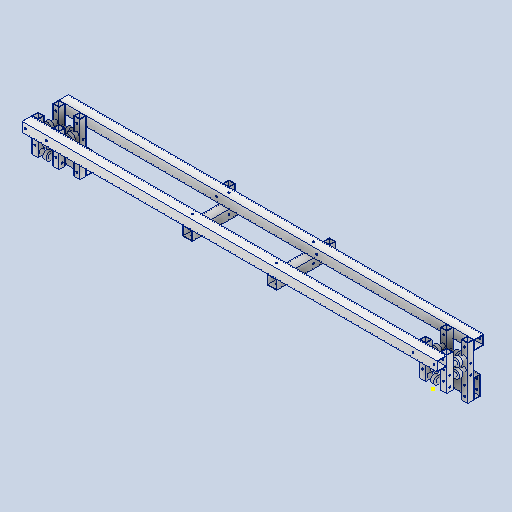
# Autodesk Inventor part: RZvector-Srunit-v3-ASP-Base
Saved by Autodesk Inventor 2025.2 (Build 292293000, 293)
## iProperties
Created: 2024-04-13
Part Number: RZvector-Srunit-v3-ASP-Base
Material: アルミニウム 6061
Document SubType Name: Modeling
Designer: haruy
Density: 2.7 g/cm^3
Appearance: アルミニウム - フラット
Author: haruy
Autodesk Inventor part; units mm, degrees
ref_plane "YZ Plane" through (0, 0, 0) normal (1, 0, 0) x (0, 1, 0)
ref_plane "XZ Plane" through (0, 0, 0) normal (0, 1, 0) x (-1, 0, 0)
ref_plane "XY Plane" through (0, 0, 0) normal (0, 0, 1) x (1, 0, 0)
derived "RZvector-Srunit-v2-Sketch-Base.ipt"
sketch "正面から" plane through (0, 0, 0) normal (0, 0, 1) x (1, 0, 0)
  line L0 (0, 0) -> (20, 0)
  line L1 (20, 0) -> (20, 80)
  line L2 (20, 80) -> (0, 80)
  line L3 (0, 80) -> (0, 0)
  line L4 (21.5, 92) -> (31.5, 92)
  line L5 (31.5, 92) -> (31.5, 0)
  line L6 (31.5, 0) -> (21.5, 0)
  line L7 (21.5, 0) -> (21.5, 92)
  line L8 (-11.5, 62) -> (-1.5, 62)
  line L9 (-1.5, 62) -> (-1.5, 0)
  line L10 (-1.5, 0) -> (-11.5, 0)
  line L11 (-11.5, 0) -> (-11.5, 62)
  line L12 (-1.5, 24.5) -> (21.5, 24.5)
  line L13 (21.5, 24.5) -> (21.5, 18.5)
  line L14 (21.5, 18.5) -> (-1.5, 18.5)
  line L15 (-1.5, 18.5) -> (-1.5, 24.5)
  line L16 (7.5, 28) -> (12.5, 28)
  line L17 (12.5, 28) -> (12.5, 15)
  line L18 (12.5, 15) -> (7.5, 15)
  line L19 (7.5, 15) -> (7.5, 28)
  circle A0 centre (26.5, 29.5) radius 3
  line L20 (31.5, 15) -> (-189.7387, 15)
  line L21 (-189.7387, 15) -> (-189.7387, 0)
  line L22 (-189.7387, 0) -> (31.5, 0)
  line L23 (31.5, 0) -> (31.5, 15)
  line L24 (31.5, 92) -> (41.5, 92)
  line L25 (41.5, 92) -> (41.5, 62)
  line L26 (41.5, 62) -> (31.5, 62)
  line L27 (31.5, 62) -> (31.5, 92)
  circle A1 centre (26.5, 29.5) radius 6.5
  circle A2 centre (-6.5, 29.5) radius 6.5
  line L28 (21.5, 23) -> (31.5, 23)
  line L29 (21.5, 20) -> (31.5, 20)
  circle A3 centre (26.5, 29.5) radius 1.5
  circle A4 centre (-6.5, 29.5) radius 3
  circle A5 centre (-6.5, 29.5) radius 1.5
  line L30 (-1.5, 40.5) -> (21.5, 40.5)
  line L31 (21.5, 40.5) -> (21.5, 34.5)
  line L32 (21.5, 34.5) -> (-1.5, 34.5)
  line L33 (-1.5, 34.5) -> (-1.5, 40.5)
  line L34 (7.5, 44) -> (12.5, 44)
  line L35 (12.5, 44) -> (12.5, 31)
  line L36 (12.5, 31) -> (7.5, 31)
  line L37 (7.5, 31) -> (7.5, 44)
  circle A6 centre (-6.5, 45.5) radius 6.5
  circle A7 centre (-6.5, 45.5) radius 3
  circle A8 centre (-6.5, 45.5) radius 1.5
  line L38 (-11.5, 62) -> (31.5, 62)
  line L39 (31.5, 62) -> (31.5, 52)
  line L40 (31.5, 52) -> (-11.5, 52)
  line L41 (-11.5, 52) -> (-11.5, 62)
  circle A9 centre (26.5, 45.5) radius 6.5
  circle A10 centre (26.5, 45.5) radius 3
  circle A11 centre (26.5, 45.5) radius 1.5
  line L42 (31.5, 47) -> (31.5, 62)
  line L43 (-145, 64.5) -> (31.5, 64.5)
  line L44 (31.5, 64.5) -> (31.5, 49.5)
  line L45 (31.5, 49.5) -> (-145, 49.5)
  line L46 (-145, 49.5) -> (-145, 64.5)
  line L47 (31.5, 52) -> (-295, 52)
  line L48 (-295, 52) -> (-295, 67)
  line L49 (-295, 67) -> (31.5, 67)
  line L50 (31.5, 67) -> (31.5, 52)
  line L51 (-11.5, 15) -> (31.5, 15)
  line L52 (31.5, 15) -> (31.5, -15)
  line L53 (31.5, -15) -> (-11.5, -15)
  line L54 (-11.5, -15) -> (-11.5, 15)
  line L55 (21.5, 0) -> (21.5, -15)
  line L56 (-1.5, 0) -> (-1.5, -15)
  line L57 (-1.5, 62) -> (-1.5, 67)
  line L58 (-11.5, 62) -> (-11.5, 67)
  point P0 (-6.5, 7.5)
  point P1 (26.5, 7.5)
  point P2 (-6.5, 59.5)
  point P3 (10, 57)
  point P4 (26.5, 59.5)
  point P5 (-1.5, 52)
  point P6 (-1.5, 62)
  point P7 (-135, 56.75)
  point P8 (-1.5, 49.5)
  point P9 (-1.5, 49.6533)
  point P10 (-1.3765, 49.5)
  point P11 (-6.5, -7.5)
  point P12 (26.5, -7.5)
  point P13 (31.5, 0)
  point P14 (21.5, 67)
  point P15 (31.5, 67)
  point P16 (21.5, 15)
  point P17 (31.5, 0)
  point P18 (-1.5, 15)
  dimension "d1" = 7.5
  dimension "d2" = 7.5
  dimension "d3" = 5
  dimension "d4" = 5
  dimension "d6" = 5
  dimension "d7" = 10
  dimension "d8" = 5
  dimension "d10" = 5
  dimension "d90" = 176.5
  dimension "d91" = 15
  dimension "d92" = 2.5
  dimension "d93" = 0
  dimension "d94" = 7.25
  dimension "d95" = 10
  dimension "d179" = 15
  dimension "d180" = 326.5
  dimension "d181" = 7.5
  dimension "d182" = 7.5
  dimension "d183" = 43
  dimension "d184" = 30
  measures "d1" distance from line of point (-6.5, 7.5) L10
  measures "d2" distance from line of point (26.5, 7.5) L6
  measures "d3" distance from line of point (-6.5, 7.5) L9
  measures "d4" distance from line of point (26.5, 7.5) L7
  measures "d6" distance from line of point (-6.5, 59.5) L9
  measures "d7" distance from line of point (10, 57) L3
  measures "d8" distance from line of point (10, 57) L40
  measures "d10" distance from line of point (26.5, 59.5) L5
  measures "d90" distance of L44.end L45.end
  measures "d91" distance of L43.end L44.end
  measures "d92" distance between parallel lines of L8 L43
  measures "d93" distance between parallel lines of L5 L44
  measures "d94" distance from line of point (-135, 56.75) L45
  measures "d95" distance from line of L46 point (-135, 56.75)
  measures "d179" distance of L47.end L48.end
  measures "d180" distance between parallel lines of L27 L48
  measures "d181" distance from line of point (-6.5, 59.5) L47
  measures "d182" distance from line of point (26.5, 59.5) L40
  measures "d183" distance of L52.end L53.end
  measures "d184" distance of L51.end L52.end
sketch "横から" plane through (0, 0, 0) normal (1, 0, 0) x (0, 1, 0)
  line L0 (0, 0) -> (200, 0)
  line L1 (200, 0) -> (200, -20)
  line L2 (200, -20) -> (0, -20)
  line L3 (0, -20) -> (0, 0)
  circle A0 centre (21.5, 6.5) radius 6.5
  circle A1 centre (21.5, -26.5) radius 6.5
  line L4 (15, 26.5) -> (0, 26.5)
  line L5 (0, 26.5) -> (0, 11.5)
  line L6 (0, 11.5) -> (15, 11.5)
  line L7 (15, 11.5) -> (15, 26.5)
  line L8 (15, -31.5) -> (0, -31.5)
  line L9 (0, -31.5) -> (0, -46.5)
  line L10 (0, -46.5) -> (15, -46.5)
  line L11 (15, -46.5) -> (15, -31.5)
  line L12 (62, 11.5) -> (0, 11.5)
  line L13 (0, 11.5) -> (0, 1.5)
  line L14 (0, 1.5) -> (62, 1.5)
  line L15 (62, 1.5) -> (62, 11.5)
  line L16 (62, -21.5) -> (0, -21.5)
  line L17 (0, -21.5) -> (0, -31.5)
  line L18 (0, -31.5) -> (62, -31.5)
  line L19 (62, -31.5) -> (62, -21.5)
  line L20 (36, -7.5) -> (23, -7.5)
  line L21 (23, -7.5) -> (23, -12.5)
  line L22 (23, -12.5) -> (36, -12.5)
  line L23 (36, -12.5) -> (36, -7.5)
  line L24 (92, 11.5) -> (62, 11.5)
  line L25 (62, 11.5) -> (62, -31.5)
  line L26 (62, -31.5) -> (92, -31.5)
  line L27 (92, -31.5) -> (92, 11.5)
  circle A2 centre (37.5, 6.5) radius 6.5
  circle A3 centre (37.5, -26.5) radius 6.5
  line L28 (52, -7.5) -> (39, -7.5)
  line L29 (39, -7.5) -> (39, -12.5)
  line L30 (39, -12.5) -> (52, -12.5)
  line L31 (52, -12.5) -> (52, -7.5)
  line L32 (52, 11.5) -> (52, -31.5)
  point P0 (62, -26.5)
extrude "押し出し1" add sketch "正面から" along normal blind 10 contours L10 L11 L20 L9 | L20 L11 A2 L9 | L11 A2 L9 | A2 L11 A6 L9 | L11 L45 L9 A6 | L11 A6 L9 L45 | L11 L40 A6 | A6 L40 L9 | L11 L8 L9 L40 | A4 | A5 | A7 | A8
extrude "押し出し2" add sketch "正面から" along normal blind 10 separate body contours L7 L20 L5 L6 | L7 L29 L5 L20 | L7 A1 L28 | L7 L28 L5 L29 | A1 L5 L7 | L7 A9 L5 A1 | L28 A1 L5 | A9 L7 L45 L5 | A9 L5 L45 L7 | L7 L40 A9 | A9 L40 L5 | L7 L38 L5 L40 | L7 L43 L5 L38 | L7 L49 L5 L43 | L7 L4 L5 L49 | A0 | A3 | A10 | A11
ref_plane "作業平面1" through (-1.5, 0, -23) normal (0, 0, -1) x (-1, 0, 0)
extrude "押し出し3" add sketch "正面から" against normal blind 10 from surface at -23 separate body contours L10 L11 L20 L9 | L20 L11 A2 L9 | L11 A2 L9 | A2 L11 A6 L9 | L11 L45 L9 A6 | L11 A6 L9 L45 | L11 L40 A6 | A6 L40 L9 | A4 | A5 | A7 | A8
extrude "押し出し4" add sketch "正面から" against normal blind 10 from surface at -23 separate body contours L7 L20 L5 L6 | L7 L29 L5 L20 | L7 A1 L28 | L7 L28 L5 L29 | A1 L5 L7 | L7 A9 L5 A1 | L28 A1 L5 | A9 L7 L45 L5 | A9 L5 L45 L7 | L7 L40 A9 | A9 L40 L5 | L7 L38 L5 L40 | L7 L43 L5 L38 | L7 L49 L5 L43 | L7 L4 L5 L49 | A0 | A3 | A10 | A11
ref_plane "作業平面2" through (-11.5, 0, 10) normal (0, 0, 1) x (1, 0, 0)
extrude "押し出し5" add sketch "正面から" along normal blind 15 from surface at 10 separate body contours L45 A6 L11 | L11 A6 L9 L45 | L45 L46 L47 L11 A6 | L45 A6 L9 L40 L3 | L3 L40 L1 L45 | L45 L9 A6 | L11 L40 A6 | L1 L40 L7 A9 L45 | A9 L7 L45 | L40 L9 L38 L3 | L3 L38 L1 L40 | A6 L40 L9 | L47 L46 L43 L58 L11 | L11 L8 L9 L40 | L1 L38 L7 L40 | A9 L5 L45 L7 | L7 L40 A9 | A9 L40 L5 | L38 L57 L43 L3 | L3 L43 L1 L38 | L58 L43 L57 L8 | L1 L43 L7 L38 | L7 L38 L5 L40 | L7 L43 L5 L38 picked at (-11.5139, 49.5853) picked at (-6.5, 50.3333) picked at (-1.4861, 49.5853) picked at (21.4861, 49.5853) picked at (26.5, 50.3333)
sketch "スケッチ3" plane through (31.5, 0, 0) normal (1, 0, 0) x (0, 0, -1)
  line L0 (-10, 92) -> (-10, 0) projected
  line L1 (-10, 92) -> (33, 92)
  line L2 (33, 92) -> (33, 62)
  line L3 (33, 62) -> (-10, 62)
  line L4 (-10, 62) -> (-10, 92)
  point P0 (0, 0)
  dimension "d23" = 43
  dimension "d24" = 30
  constraints: 8 end point, 2 parallel, 1 horizontal, 1 perpendicular
  measures "d23" distance of L2.end L3.end
  measures "d24" distance of L1.end L2.end
extrude "押し出し6" add sketch "スケッチ3" along normal blind 10 separate body
shell "シェル1" thickness 1 removed faces 11 at (-4.8333, 52, -26.3333) at (-8.1667, 0, -26.3333) at (24.8333, 0, -26.3333) at (-8.1667, 0, 3.3333) at (24.8333, 0, 3.3333) at (31.5, 54.5, 20) at (28.1667, 92, 6.6667) at (28.1667, 92, -26.3333) at (38.1667, 72, 10) at (34.8333, 72, -33) at (-4.8333, 62, 3.3333) bodies 3 4 1 2 5 6
hole "穴1" at (-6.5, 7.5, 0) at (26.5, 7.5, 0) at (-6.5, 59.5, 0) at (10, 57, 0) at (26.5, 59.5, 0) at (26.5, 29.5, 0) at (-6.5, 29.5, 0) at (-6.5, 45.5, 0) at (26.5, 45.5, 0) at (-135, 56.75, 0) direction (0, 0, 1) diameter 3 end through all both bodies 2 1 5 3
hole "穴2" at (26.5, 45.5, 0) at (26.5, 29.5, 0) at (26.5, 7.5, 0) direction (0, 0, -1) diameter 3 end through all bodies 4
sketch "スケッチ4" plane through (41.5, 0, 0) normal (1, 0, 0) x (0, 0, -1)
  line L0 (-10, 92) -> (-10, 62) projected
  line L1 (33, 62) -> (33, 92) projected
  line L2 (33, 92) -> (-10, 92) projected
  line L3 (0, 0) -> (-10, 0) projected
  line L4 (33, 0) -> (23, 0) projected
  line L5 (-10, 0) -> (-10, 92) projected
  line L6 (23, 0) -> (23, 92) projected
  line L7 (-10, 62) -> (33, 62) projected
  point P0 (-5, 84.5)
  point P1 (28, 84.5)
  point P2 (-5, 21.5)
  point P3 (-5, 37.5)
  point P4 (28, 37.5)
  point P5 (28, 21.5)
  point P6 (-5, 69.5)
  point P7 (28, 69.5)
  dimension "d42" = 5
  dimension "d43" = 5
  dimension "d44" = 7.5
  dimension "d45" = 7.5
  dimension "d46" = 21.5
  dimension "d47" = 21.5
  dimension "d48" = 16
  dimension "d49" = 16
  dimension "d50" = 5
  dimension "d51" = 5
  dimension "d52" = 5
  dimension "d53" = 5
  dimension "d84" = 5
  dimension "d85" = 5
  dimension "d86" = 7.5
  dimension "d87" = 7.5
  measures "d42" distance from line of point (-5, 84.5) L0
  measures "d43" distance from line of L1 point (28, 84.5)
  measures "d44" distance from line of point (-5, 84.5) L2
  measures "d45" distance from line of L2 point (28, 84.5)
  measures "d46" distance from line of point (-5, 21.5) L3
  measures "d47" distance from line of point (28, 21.5) L4
  measures "d48" distance of point (-5, 37.5) point (-5, 21.5)
  measures "d49" distance of point (28, 37.5) point (28, 21.5)
  measures "d50" distance from line of point (-5, 21.5) L5
  measures "d51" distance from line of point (-5, 37.5) L5
  measures "d52" distance from line of point (28, 21.5) L6
  measures "d53" distance from line of point (28, 37.5) L6
  measures "d84" distance from line of L0 point (-5, 69.5)
  measures "d85" distance from line of L1 point (28, 69.5)
  measures "d86" distance from line of point (-5, 69.5) L7
  measures "d87" distance from line of point (28, 69.5) L7
hole "穴3" at (41.5, 84.5, 5) at (41.5, 84.5, -28) at (41.5, 21.5, 5) at (41.5, 37.5, 5) at (41.5, 37.5, -28) at (41.5, 21.5, -28) at (41.5, 69.5, 5) at (41.5, 69.5, -28) direction (-1, 0, 0) diameter 3 end through all bodies 6 2 4 1 3
extrude "押し出し7" add sketch "正面から" against normal up to surface (23 mm away) separate body contours A0 | A4 | A7 | A10
sketch "スケッチ5" plane through (21.5, 0, -33) normal (-1, 0, 0) x (0, 0, 1)
  circle A0 centre (5, 37.5) radius 1.5 projected
  circle A1 centre (5, 37.5) radius 3
  circle A2 centre (5, 37.5) radius 1.5
  circle A3 centre (5, 21.5) radius 1.5 projected
  circle A4 centre (5, 21.5) radius 3
  circle A5 centre (5, 21.5) radius 1.5
  circle A6 centre (38, 37.5) radius 1.5 projected
  circle A7 centre (38, 37.5) radius 3
  circle A8 centre (38, 21.5) radius 1.5 projected
  circle A9 centre (38, 21.5) radius 3
  circle A10 centre (38, 21.5) radius 1.5
  circle A11 centre (38, 37.5) radius 1.5
  circle A12 centre (5, 37.5) radius 6.5
  circle A13 centre (5, 21.5) radius 6.5
  circle A14 centre (38, 21.5) radius 6.5
  circle A15 centre (38, 37.5) radius 6.5
  point P0 (33, 0)
  dimension "d63" = 6
  dimension "d64" = 3
  dimension "d65" = 6
  dimension "d66" = 3
  dimension "d67" = 6
  dimension "d68" = 6
  dimension "d69" = 3
  dimension "d70" = 3
  dimension "d76" = 13
  dimension "d77" = 13
  dimension "d78" = 13
  dimension "d79" = 13
  constraints: 12 centre point, 12 coincident
  measures "d63" diameter of A1
  measures "d64" diameter of A2
  measures "d65" diameter of A4
  measures "d66" diameter of A5
  measures "d67" diameter of A7
  measures "d68" diameter of A9
  measures "d69" diameter of A10
  measures "d70" diameter of A11
  measures "d76" diameter of A12
  measures "d77" diameter of A13
  measures "d78" diameter of A14
  measures "d79" diameter of A15
extrude "押し出し8" add sketch "スケッチ5" along normal up to surface (23 mm away) separate body contours A1 | A4 | A7 | A9
ref_plane "作業平面3" through (-1.5, 0, -11.5) normal (0, 0, -1) x (-1, 0, 0)
extrude "押し出し9" add sketch "正面から" along normal mid plane 5 from surface at -11.5 separate body contours A2 L9 | A2 L11 | L11 A2 L9 | A1 L7 | A1 L5 L7 | A6 L45 L11 | L11 L45 L9 A6 | A1 L5 | A6 L9 L45 | L45 A6 L11 | L11 A6 L9 L45 | A9 L45 L7 | A9 L7 L45 L5 | L5 A9 | L45 L9 A6 | A9 L7 L45 | A9 L5 L45 L7
ref_plane "作業平面4" through (10, 0, 0) normal (-1, 0, 0) x (0, 0, 1)
extrude "押し出し10" add sketch "スケッチ5" along normal mid plane 5 from surface at 11.5 separate body contours A12 | A13 | A14 | A15
ref_plane "作業平面5" through (-295, 0, -33) normal (-1, 0, 0) x (0, 0, 1)
ref_plane "作業平面6" through (-11.5, 0, -11.5) normal (0, 0, 1) x (1, 0, 0)
sketch "スケッチ14" plane through (31.5, 92, 0) normal (0, 0, -1) x (-1, 0, 0)
  point P0 (31.5, -92)
extrude "押し出し15" add sketch "正面から" along normal blind 10 contours L6 L52 L53 L55 bodies 2
extrude "押し出し16" add sketch "正面から" along normal blind 10 contours L56 L53 L54 L10 bodies 1
extrude "押し出し17" add sketch "正面から" against normal blind 10 from surface at -23 contours L6 L52 L53 L55 bodies 4
extrude "押し出し18" add sketch "正面から" against normal blind 10 from surface at -23 contours L56 L53 L54 L10 bodies 3
extrude "押し出し19" cut sketch "正面から" along normal blind 10 contours L7 L4 L5 L49 bodies 2
extrude "押し出し20" add sketch "正面から" along normal blind 10 contours L58 L43 L57 L8 | L58 L49 L57 L43 bodies 1
extrude "押し出し21" cut sketch "正面から" against normal blind 10 from surface at -23 contours L7 L4 L5 L49 bodies 4
extrude "押し出し22" add sketch "正面から" against normal blind 10 from surface at -23 contours L11 L8 L9 L40 | L58 L43 L57 L8 | L58 L49 L57 L43 bodies 3
shell "シェル3" thickness 1 removed faces 12 at (-8.1667, -15, 3.3333) at (-4.8333, 67, 3.3333) at (25.1667, 0, 6.3333) at (24.8333, -15, 6.6667) at (-4.8333, 67, -26.3333) at (-8.1667, -15, -26.3333) at (-5.1667, 0, -26.6667) at (-7.8333, 52, -26.6667) at (24.8333, -15, -26.3333) at (27.8333, 0, -26.6667) at (-5.1667, 62, 6.3333) at (-7.8333, 0, 6.3333) bodies 2 4 3 1
extrude "押し出し23" cut sketch "正面から" along normal blind 10 contours L7 L20 L5 L6 | L6 L52 L53 L55 bodies 2
extrude "押し出し24" cut sketch "正面から" along normal blind 10 contours L10 L11 L20 L9 | L56 L53 L54 L10 bodies 1
hole "穴10" at (26.5, 59.5, 0) at (-6.5, 59.5, 0) at (26.5, -7.5, 0) at (-6.5, -7.5, 0) direction (0, 0, -1) diameter 3 end through all bodies 4 3
ref_plane "作業平面7" through (-295, -15, -23) normal (1, 0, 0) x (0, 0, -1)
extrude "押し出し25" add sketch "正面から" along normal blind 15 from surface at 10 separate body contours L40 L9 L38 L3 | L3 L38 L1 L40 | L47 L46 L43 L58 L11 | L11 L8 L9 L40 | L47 L48 L49 L58 L43 L46 | L1 L38 L7 L40 | L38 L57 L43 L3 | L3 L43 L1 L38 | L58 L43 L57 L8 | L1 L43 L7 L38 | L7 L38 L5 L40 | L43 L57 L49 L3 | L3 L49 L1 L43 | L58 L49 L57 L43 | L1 L49 L7 L43 | L7 L43 L5 L38 | L7 L49 L5 L43
shell "シェル4" thickness 1 removed faces 2 at (31.5, 57, 20) at (-295, 62, 15) bodies 11
hole "穴11" at (26.5, 59.5, 0) at (-6.5, 59.5, 0) direction (0, 0, 1) diameter 3 end through all both bodies 11
mirror "ミラー3" about plane through (-11.5, 0, -11.5) normal (0, 0, 1) bodies 11
extrude "押し出し26" add sketch "正面から" against normal blind 10 from surface at -33 separate body contours L3 L20 L18 L1 L0 | L22 L9 L20 L3 | L0 L22 L55 L53 L56 | L1 L20 L7 L22 | L10 L11 L20 L9 | L56 L53 L54 L10 | L7 L20 L5 L6 | L6 L52 L53 L55
shell "シェル5" thickness 1 removed faces 4 at (31.5, 5, -39.6667) at (31.5, -10, -36.3333) at (-11.5, -5, -36.3333) at (-11.5, 10, -36.3333) bodies 12
hole "穴12" at (26.5, 7.5, 0) at (26.5, -7.5, 0) at (-6.5, 7.5, 0) at (-6.5, -7.5, 0) direction (0, 0, -1) diameter 3 end through all bodies 12
mirror "ミラー4" about plane through (-295, -15, -23) normal (1, 0, 0) bodies 1 3 12 4 2 9 7 8 10 11
sketch "スケッチ15" plane through (31.5, 67, 25) normal (0, 1, 0) x (1, 0, 0)
  line L0 (0, 0) -> (-653, 0) projected
  line L1 (-326.5, 0) -> (-326.5, 73)
  line L2 (-653, 73) -> (0, 73) projected
  line L3 (-274, 0) -> (-294, 0)
  line L4 (-294, 0) -> (-294, 73) construction
  line L5 (-294, 73) -> (-274, 73)
  line L6 (-274, 73) -> (-274, 0) construction
  line L7 (-252.5, 0) -> (-267.5, 0)
  line L8 (-267.5, 0) -> (-267.5, 73)
  line L9 (-267.5, 73) -> (-252.5, 73)
  line L10 (-252.5, 73) -> (-252.5, 0)
  line L11 (-267.5, 73) -> (-252.5, 73)
  line L12 (-252.5, 73) -> (-252.5, 83)
  line L13 (-252.5, 83) -> (-267.5, 83)
  line L14 (-267.5, 83) -> (-267.5, 73)
  line L15 (-252.5, 73) -> (-242.5, 73)
  line L16 (-242.5, 73) -> (-242.5, 83)
  line L17 (-242.5, 83) -> (-252.5, 83)
  line L18 (-252.5, 83) -> (-252.5, 73)
  line L19 (0, 58) -> (-653, 58) projected
  point P0 (-31.5, 25)
  point P1 (-260, 65.5)
  point P2 (-260, 7.5)
  point P3 (-267.5, 0)
  point P4 (-393, 65.5)
  point P5 (-393, 7.5)
  dimension "d234" = 20
  dimension "d235" = 0
  dimension "d236" = 52.5
  dimension "d237" = 15
  dimension "d238" = 0
  dimension "d240" = 59
  dimension "d241" = 15
  dimension "d242" = 10
  dimension "d243" = 10
  dimension "d244" = 10
  dimension "d245" = 7.5
  dimension "d246" = 7.5
  dimension "d247" = 7.5
  dimension "d248" = 7.5
  constraints: 34 end point, 8 parallel, 4 horizontal, 4 perpendicular, 2 midpoint, 2 point on line, 2 symmetric about line
  measures "d234" distance of L4.end L5.end
  measures "d235" distance between parallel lines of L2 L5
  measures "d236" distance between parallel lines of L1 L6
  measures "d237" distance of L8.end L9.end
  measures "d238" distance between parallel lines of L2 L9
  measures "d240" distance between parallel lines of L1 L8
  measures "d241" distance of L13.end L12.end
  measures "d242" distance of L12.end L11.end
  measures "d243" distance of L17.end L16.end
  measures "d244" distance of L16.end L15.end
  measures "d245" distance from line of point (-260, 7.5) L0
  measures "d246" distance from line of point (-260, 7.5) L8
  measures "d247" distance from line of L19 point (-260, 65.5)
  measures "d248" distance from line of point (-260, 65.5) L8
extrude "押し出し27" add sketch "スケッチ15" against normal blind 15 from surface at -15 separate body contours L0 L8 L19 L10 | L19 L8 L2 L10 | L2 L14 L13 L12
extrude "押し出し28" add sketch "スケッチ15" against normal up to surface (30 mm away) separate body contours L12 L17 L16 L2
shell "シェル6" thickness 1 removed faces 4 at (-231, 42, 25) at (-226, 42, -58) at (-217.6667, 67, -54.6667) at (-217.6667, 37, -54.6667) bodies 13 14
hole "穴13" at (-228.5, 67, 17.5) at (-228.5, 67, -40.5) at (-361.5, 67, 17.5) at (-361.5, 67, -40.5) direction (0, -1, 0) diameter 3 end through all bodies 11 13
sketch "スケッチ16" plane through (-211, 67, -48) normal (1, 0, 0) x (0, 0, -1)
  line L0 (0, -30) -> (10, -30) projected
  line L1 (10, 0) -> (10, -30) projected
  point P0 (-48, -67)
  point P1 (5, -22.5)
  dimension "d261" = 7.5
  dimension "d262" = 5
  measures "d261" distance from line of point (5, -22.5) L0
  measures "d262" distance from line of L1 point (5, -22.5)
hole "穴14" at (-211, 44.5, -53) direction (-1, 0, 0) diameter 3 end through all bodies 14 13
sketch "スケッチ17" plane through (-211, 67, -58) normal (0, 0, -1) x (-1, 0, 0)
  line L0 (0, 0) -> (10, 0) projected
  line L1 (0, 0) -> (0, -30) projected
  point P0 (-211, -67)
  point P1 (5, -7.5)
  dimension "d270" = 7.5
  dimension "d271" = 5
  measures "d270" distance from line of L0 point (5, -7.5)
  measures "d271" distance from line of point (5, -7.5) L1
hole "穴15" at (-216, 59.5, -58) direction (0, 0, 1) diameter 3 depth 30 tip angle 118 bodies 14 11
sketch "スケッチ18" plane through (-221, 37, -58) normal (1, 0, 0) x (0, 0, -1)
  line L0 (-83, 0) -> (-83, 15) projected
  line L1 (-83, 0) -> (0, 0) projected
  point P0 (-58, -37)
  point P1 (-68, 7.5)
  point P2 (-25, 7.5)
  dimension "d279" = 15
  dimension "d280" = 43
  dimension "d281" = 7.5
  dimension "d282" = 7.5
  measures "d279" distance from line of point (-68, 7.5) L0
  measures "d280" distance of point (-25, 7.5) point (-68, 7.5)
  measures "d281" distance from line of point (-68, 7.5) L1
  measures "d282" distance from line of point (-25, 7.5) L1
hole "穴16" at (-221, 44.5, 10) at (-221, 44.5, -33) direction (-1, 0, 0) diameter 3 depth 30 tip angle 118 bodies 13
mirror "ミラー5" about plane through (-295, -15, -23) normal (1, 0, 0) bodies 13 14
sketch "スケッチ19" plane through (31.5, 52, -33) normal (0, 0, 1) x (1, 0, 0)
  circle A0 centre (-405.5, 7.5) radius 1.5 projected
  point P0 (-31.5, -52)
  constraints: 1 coincident
hole "穴17" at (-374, 59.5, -33) direction (0, 0, -1) diameter 3 end through all bodies 11
equation "\"d246\" = d245"
equation "\"d282\" = d281"
